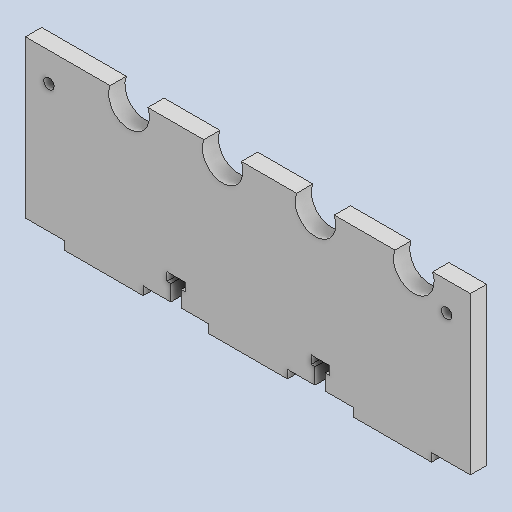
# Autodesk Inventor part: Carcasa_CajaR_Lateral1
Saved by Autodesk Inventor 2022 (Build 260153000, 153)
## iProperties
Created: 2022-02-21
Part Number: Carcasa_CajaR_Lateral1
Material: Generic
Document SubType Name: Modeling
Designer: katha
Density: 1 g/cm^3
Appearance: Default
Author: katha
Autodesk Inventor part; units mm, degrees
ref_plane "YZ Plane" through (0, 0, 0) normal (1, 0, 0) x (0, 1, 0)
ref_plane "XZ Plane" through (0, 0, 0) normal (0, 1, 0) x (-1, 0, 0)
ref_plane "XY Plane" through (0, 0, 0) normal (0, 0, 1) x (1, 0, 0)
sketch "Sketch1" plane through (0, 0, 0) normal (0, 0, 1) x (1, 0, 0)
  circle A0 centre (0.15, -0.0866) radius 7.5 projected
  circle A1 centre (35.6226, -0.0866) radius 7.5 projected
  line L0 (-37.4458, 2.8981) -> (-34.0994, 2.8981) projected
  line L1 (-39.119, 0) -> (-37.4458, 2.8981) projected
  line L2 (-37.4458, -2.8981) -> (-39.119, 0) projected
  line L3 (-34.0994, -2.8981) -> (-37.4458, -2.8981) projected
  line L4 (-32.4262, 0) -> (-34.0994, -2.8981) projected
  line L5 (-34.0994, 2.8981) -> (-32.4262, 0) projected
  line L6 (71.5994, 2.8981) -> (74.9458, 2.8981) projected
  line L7 (69.9262, 0) -> (71.5994, 2.8981) projected
  line L8 (71.5994, -2.8981) -> (69.9262, 0) projected
  line L9 (74.9458, -2.8981) -> (71.5994, -2.8981) projected
  line L10 (76.619, 0) -> (74.9458, -2.8981) projected
  line L11 (74.9458, 2.8981) -> (76.619, 0) projected
  line L12 (94.8132, 2.8981) -> (94.8132, -57.1019)
  line L13 (-75.1868, -57.1019) -> (-75.1868, 2.8981)
  line L14 (-75.1868, 2.8981) -> (94.8132, 2.8981)
  circle A2 centre (-35.6226, -0.0866) radius 7.5 projected
  circle A3 centre (73.2223, -0.0862) radius 7.5 projected
  circle A4 centre (-35.6226, -0.0866) radius 7.8
  circle A5 centre (0.15, -0.0866) radius 7.8
  circle A6 centre (35.6226, -0.0866) radius 7.8
  circle A7 centre (73.2223, -0.0862) radius 7.8
  circle A8 centre (85.8132, -8.0862) radius 2
  line L15 (73.2223, -0.0862) -> (73.2223, 6.7764) construction
  circle A9 centre (-66.1868, -8.0866) radius 2
  line L16 (95, -57.1019) -> (-75.1868, -57.1019)
  line L17 (-60.1868, -57.1019) -> (-30.1868, -57.1019)
  line L18 (-30.1868, -57.1019) -> (-30.1868, -60.3019)
  line L19 (-30.1868, -60.3019) -> (-60.1868, -60.3019)
  line L20 (-60.1868, -60.3019) -> (-60.1868, -57.1019)
  line L21 (9.9066, -57.1019) -> (9.9066, -41.5844) construction
  line L22 (9.9066, -57.1019) -> (9.9066, -60.3019)
  line L23 (9.9066, -60.3019) -> (-5.0934, -60.3019)
  line L24 (-5.0934, -60.3019) -> (-5.0934, -57.1019)
  line L25 (50, -57.1019) -> (50, -60.3019)
  line L26 (50, -60.3019) -> (80, -60.3019)
  line L27 (80, -60.3019) -> (80, -57.1019)
  line L28 (9.9066, -60.3019) -> (24.9066, -60.3019)
  line L29 (24.9066, -60.3019) -> (24.9066, -57.1019)
  point P0 (0, 0)
  point P1 (80.4289, 2.8981)
  point P2 (66.0158, 2.8981)
  point P3 (42.8289, 2.8981)
  point P4 (28.4162, 2.8981)
  point P5 (7.3564, 2.8981)
  point P6 (-7.0564, 2.8981)
  point P7 (-28.4162, 2.8981)
  point P8 (-42.8289, 2.8981)
  point P9 (94.8132, -57.1019)
  point P10 (-30.1868, -57.1019)
  point P11 (24.9066, -57.1019)
  point P12 (50, -57.1019)
  point P13 (80, -57.1019)
  dimension "d2" = 170
  dimension "d4" = 0.3
  dimension "d5" = 0.3
  dimension "d6" = 0.3
  dimension "d7" = 0.3
  dimension "d17" = 4
  dimension "d19" = 8
  dimension "d24" = 9
  dimension "d42" = 60
  dimension "d43" = 30
  dimension "d44" = 3.2
  dimension "d45" = 15
  dimension "d46" = 75.1868
  dimension "d47" = 94.8132
  dimension "d48" = 9
  dimension "d49" = 8
  dimension "d50" = 4
  dimension "d51" = 3.2
  dimension "d52" = 15
  dimension "d53" = 25.0934
  constraints: 36 end point, 6 centre point, 6 symmetric about line, 5 perpendicular, 3 parallel, 2 horizontal, 2 point on line, 2 vertical, 1 coincident, 1 collinear, 1 midpoint
  measures "d2" distance of L13.start L12.end
  measures "d4" radial gap between concentric circles of A2 A4
  measures "d5" radial gap between concentric circles of A0 A5
  measures "d6" radial gap between concentric circles of A1 A6
  measures "d7" radial gap between concentric circles of A3 A7
  measures "d17" diameter of A8
  measures "d19" vertical distance of A8.centre A3.centre
  measures "d24" distance from line of L12 A8.centre
  measures "d42" distance between parallel lines of L16 L14
  measures "d43" distance of L18.end L19.end
  measures "d44" distance of L17.end L18.end
  measures "d45" distance between parallel lines of L20 L13
  measures "d46" distance from line of L13 point (0, 0)
  measures "d47" distance from line of L12 point (0, 0)
  measures "d48" distance from line of L13 A9.centre
  measures "d49" vertical distance of A9.centre A2.centre
  measures "d50" diameter of A9
  measures "d51" distance of L21.start L22.end
  measures "d52" distance of L22.end L23.end
  measures "d53" distance between parallel lines of L24 L18
extrude "Extrusion3" add sketch "Sketch1" along normal blind 0.1 and the other way blind 6.1 contours L14 A6 A7 L12 L16 L13 A4 A5 | L16 L18 L19 L20 | L27 L26 L25 L16 | L16 L22 L23 L24 | L16 L29 L28 L22
sketch "Sketch2" plane through (0, 0, 0.1) normal (0, 0, 1) x (1, 0, 0)
  line L0 (-5.0934, -60.3019) -> (24.9066, -60.3019) projected
  line L1 (24.9066, -60.3019) -> (-5.0934, -60.3019) projected
  line L2 (9.9066, -60.3019) -> (9.9066, -41.2301) construction
  line L3 (-30.1868, -57.1019) -> (-5.0934, -57.1019) projected
  line L4 (-17.6401, -57.1019) -> (-17.6401, -48.823) construction
  line L5 (-19.6401, -57.1019) -> (-15.6401, -57.1019)
  line L6 (-15.6401, -57.1019) -> (-15.6401, -51.0019)
  line L7 (-19.6401, -51.0019) -> (-19.6401, -57.1019)
  line L8 (-17.6401, -51.0019) -> (-14.1401, -51.0019)
  line L9 (-14.1401, -51.0019) -> (-14.1401, -47.8019)
  line L10 (-19.6401, -51.0019) -> (-15.6401, -51.0019)
  line L11 (-17.6401, -51.0019) -> (-21.1401, -51.0019)
  line L12 (-21.1401, -51.0019) -> (-21.1401, -47.8019)
  line L13 (-21.1401, -47.8019) -> (-14.1401, -47.8019)
  line L14 (37.4533, -57.1019) -> (37.4533, -48.823) construction
  line L15 (39.4533, -57.1019) -> (35.4533, -57.1019)
  line L16 (35.4533, -57.1019) -> (35.4533, -51.0019)
  line L17 (39.4533, -51.0019) -> (39.4533, -57.1019)
  line L18 (37.4533, -51.0019) -> (33.9533, -51.0019)
  line L19 (33.9533, -51.0019) -> (33.9533, -47.8019)
  line L20 (39.4533, -51.0019) -> (35.4533, -51.0019)
  line L21 (37.4533, -51.0019) -> (40.9533, -51.0019)
  line L22 (40.9533, -51.0019) -> (40.9533, -47.8019)
  line L23 (40.9533, -47.8019) -> (33.9533, -47.8019)
  point P0 (0, 0)
  dimension "d64" = 2
  dimension "d65" = 3.5
  dimension "d66" = 3.2
  dimension "d67" = 4
  dimension "d68" = 6.1
  dimension "d69" = 7
  constraints: 42 end point, 13 symmetric about line, 2 collinear, 2 horizontal, 2 midpoint, 2 perpendicular, 2 vertical, 1 parallel, 1 point on line
  measures "d64" distance between parallel lines of L6 L4
  measures "d65" distance of L8.start L8.end
  measures "d66" distance of L8.end L9.end
  measures "d67" distance between parallel lines of L6 L7
  measures "d68" distance between parallel lines of L5 L11
  measures "d69" distance between parallel lines of L9 L12
extrude "Extrusion4" cut sketch "Sketch2" against normal blind 7
body "Solid3"
